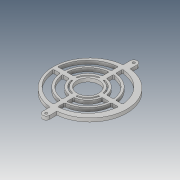
# Autodesk Inventor part: verticalThrusterCover2
Saved by Autodesk Inventor 2018 (Build 220112000, 112)
## iProperties
Created: 2020-02-09
Part Number: verticalThrusterCover2
Material: Generic
Document SubType Name: Modeling
Designer: anirudh
Density: 1 g/cm^3
Appearance: Default
Author: anirudh
Autodesk Inventor part; units mm, degrees
ref_plane "YZ Plane" through (0, 0, 0) normal (1, 0, 0) x (0, 1, 0)
ref_plane "XZ Plane" through (0, 0, 0) normal (0, 1, 0) x (-1, 0, 0)
ref_plane "XY Plane" through (0, 0, 0) normal (0, 0, 1) x (1, 0, 0)
sketch "Sketch1" plane through (0, 0, 0) normal (0, 1, 0) x (-1, 0, 0)
  circle A0 centre (0, -63.5) radius 1.75
  circle A1 centre (0, 63.5) radius 1.75
  circle A2 centre (0, -63.5) radius 1.75
  circle A3 centre (0, 63.5) radius 1.75
  arc A4 (5.08, 63.5) -> (-5.08, 63.5) centre (0, 63.5) ccw
  arc A5 (-5.08, -63.5) -> (5.08, -63.5) centre (0, -63.5) ccw
  line L0 (5.08, 63.5) -> (5.08, 53.0975)
  line L1 (5.08, -53.0975) -> (5.08, -63.5)
  line L2 (-5.08, -63.5) -> (-5.08, -53.0975)
  line L3 (-5.08, 53.0975) -> (-5.08, 63.5)
  arc A6 (-5.08, 53.0975) -> (-5.08, -53.0975) centre (0, 0) ccw
  arc A7 (5.08, -53.0975) -> (5.08, 53.0975) centre (0, 0) ccw
  arc A8 (-0.1848, -27.646) -> (6.1284, -27.646) centre (2.9718, -27.305) ccw
  line L4 (6.8199, -21.2443) -> (6.1284, -27.646)
  line L5 (-0.1848, -27.646) -> (-0.8763, -21.2443)
  line L6 (30.6178, -3.1566) -> (24.2161, -3.8481)
  line L7 (24.2161, 3.8481) -> (30.6178, 3.1566)
  arc A9 (30.6178, -3.1566) -> (30.6178, 3.1566) centre (30.2768, 0) ccw
  line L8 (6.1284, 27.646) -> (6.8199, 21.2443)
  line L9 (-0.8763, 21.2443) -> (-0.1848, 27.646)
  arc A10 (6.1284, 27.646) -> (-0.1848, 27.646) centre (2.9718, 27.305) ccw
  line L10 (-24.6742, 3.1566) -> (-18.2725, 3.8481)
  line L11 (-18.2725, -3.8481) -> (-24.6742, -3.1566)
  arc A11 (-24.6742, 3.1566) -> (-24.6742, -3.1566) centre (-24.3332, 0) ccw
  arc A12 (24.2161, 3.8481) -> (6.8199, 21.2443) centre (2.9718, 0) ccw
  arc A13 (-0.8763, 21.2443) -> (-18.2725, 3.8481) centre (2.9718, 0) ccw
  arc A14 (-18.2725, -3.8481) -> (-0.8763, -21.2443) centre (2.9718, 0) ccw
  arc A15 (6.8199, -21.2443) -> (24.2161, -3.8481) centre (2.9718, 0) ccw
  dimension "d34" = 360
  constraints: 24 end point, 24 point on circle, 16 centre point, 4 coincident, 4 vertical, 2 concentric, 33 other
extrude "Extrusion2" add sketch "Sketch1" along normal blind 5.08
sketch "Sketch3" plane through (0, 5.08, 0) normal (0, 1, 0) x (1, 0, 0)
  arc A0 (-6.8199, 21.2443) -> (-24.2161, 3.8481) centre (-2.9718, 0) ccw projected
  circle A1 centre (-2.9718, 0) radius 15.875
  circle A2 centre (-2.9718, 0) radius 38.7434
  point P0 (0, 0)
  dimension "d54" = 31.75
  constraints: 2 centre point, 2 coincident
  measures "d54" diameter of A1
extrude "Extrusion4" add sketch "Sketch3" against normal blind 5.08
sketch "Sketch4" plane through (0, 5.08, 0) normal (0, 1, 0) x (1, 0, 0)
  arc A0 (-50.0581, -3.175) -> (-6.1468, -47.0863) centre (-2.9718, 0) ccw
  arc A1 (0.2032, -47.0863) -> (44.1145, -3.175) centre (-2.9718, 0) ccw
  arc A2 (-40.0292, -3.175) -> (-6.1468, -37.0574) centre (-2.9718, 0) ccw
  arc A3 (0.2032, -37.0574) -> (34.0856, -3.175) centre (-2.9718, 0) ccw
  arc A4 (-36.8415, -3.175) -> (-6.1468, -33.8697) centre (-2.9718, 0) ccw
  arc A5 (0.2032, -33.8697) -> (30.8979, -3.175) centre (-2.9718, 0) ccw
  arc A6 (-26.7792, -3.175) -> (-6.1468, -23.8074) centre (-2.9718, 0) ccw
  arc A7 (0.2032, -23.8074) -> (20.8356, -3.175) centre (-2.9718, 0) ccw
  arc A8 (-23.5718, -3.175) -> (-6.1468, -20.6) centre (-2.9718, 0) ccw
  arc A9 (0.2032, -20.6) -> (17.6282, -3.175) centre (-2.9718, 0) ccw
  arc A10 (-21.7554, -3.175) -> (-6.1468, -18.7836) centre (-2.9718, 0) ccw
  arc A11 (0.2032, -18.7836) -> (15.8118, -3.175) centre (-2.9718, 0) ccw
  arc A12 (-21.7554, -3.175) -> (-6.1468, -18.7836) centre (-2.9718, 0) ccw
  arc A13 (0.2032, -18.7836) -> (15.8118, -3.175) centre (-2.9718, 0) ccw
  arc A14 (15.8118, 3.175) -> (0.2032, 18.7836) centre (-2.9718, 0) ccw
  arc A15 (-6.1468, 18.7836) -> (-21.7554, 3.175) centre (-2.9718, 0) ccw
  arc A16 (17.6282, 3.175) -> (0.2032, 20.6) centre (-2.9718, 0) ccw
  arc A17 (-6.1468, 20.6) -> (-23.5718, 3.175) centre (-2.9718, 0) ccw
  arc A18 (15.8118, 3.175) -> (0.2032, 18.7836) centre (-2.9718, 0) ccw
  arc A19 (-6.1468, 18.7836) -> (-21.7554, 3.175) centre (-2.9718, 0) ccw
  arc A20 (20.8356, 3.175) -> (0.2032, 23.8074) centre (-2.9718, 0) ccw
  arc A21 (-6.1468, 23.8074) -> (-26.7792, 3.175) centre (-2.9718, 0) ccw
  arc A22 (30.8979, 3.175) -> (0.2032, 33.8697) centre (-2.9718, 0) ccw
  arc A23 (-6.1468, 33.8697) -> (-36.8415, 3.175) centre (-2.9718, 0) ccw
  arc A24 (34.0856, 3.175) -> (0.2032, 37.0574) centre (-2.9718, 0) ccw
  arc A25 (-6.1468, 37.0574) -> (-40.0292, 3.175) centre (-2.9718, 0) ccw
  arc A26 (44.1145, 3.175) -> (0.2032, 47.0863) centre (-2.9718, 0) ccw
  arc A27 (-6.1468, 47.0863) -> (-50.0581, 3.175) centre (-2.9718, 0) ccw
  line L0 (-6.1468, -37.0574) -> (-6.1468, -47.0863)
  line L1 (0.2032, -37.0574) -> (0.2032, -47.0863)
  line L2 (-6.1468, -47.0863) -> (-6.1468, -37.0574)
  line L3 (-6.1468, -18.7836) -> (-6.1468, -20.6)
  line L4 (-6.1468, -23.8074) -> (-6.1468, -33.8697)
  line L5 (-6.1468, -33.8697) -> (-6.1468, -23.8074)
  line L6 (-6.1468, -20.6) -> (-6.1468, -18.7836)
  line L7 (0.2032, -18.7836) -> (0.2032, -20.6)
  line L8 (0.2032, -23.8074) -> (0.2032, -33.8697)
  line L9 (15.8118, -3.175) -> (17.6282, -3.175)
  line L10 (20.8356, -3.175) -> (30.8979, -3.175)
  line L11 (34.0856, -3.175) -> (44.1145, -3.175)
  line L12 (44.1145, 3.175) -> (34.0856, 3.175)
  line L13 (30.8979, 3.175) -> (20.8356, 3.175)
  line L14 (17.6282, 3.175) -> (15.8118, 3.175)
  line L15 (0.2032, 20.6) -> (0.2032, 18.7836)
  line L16 (0.2032, 47.0863) -> (0.2032, 37.0574)
  line L17 (0.2032, 33.8697) -> (0.2032, 23.8074)
  line L18 (-6.1468, 18.7836) -> (-6.1468, 20.6)
  line L19 (-6.1468, 23.8074) -> (-6.1468, 33.8697)
  line L20 (-6.1468, 37.0574) -> (-6.1468, 47.0863)
  line L21 (-21.7554, 3.175) -> (-23.5718, 3.175)
  line L22 (-26.7792, 3.175) -> (-36.8415, 3.175)
  line L23 (-40.0292, 3.175) -> (-50.0581, 3.175)
  line L24 (-40.0292, -3.175) -> (-50.0581, -3.175)
  line L25 (-21.7554, -3.175) -> (-23.5718, -3.175)
  line L26 (-26.7792, -3.175) -> (-36.8415, -3.175)
  constraints: 56 point on circle, 54 end point, 28 centre point, 7 coincident, 3 horizontal
extrude "Extrusion5" cut sketch "Sketch4" against normal blind 5.08
fillet "Fillet4" radius 1.27 32 edges at (-50.0581, 2.54, 3.175) (-40.0292, 2.54, 3.175) (-36.8415, 2.54, 3.175) (-26.7792, 2.54, 3.175) (-6.1468, 2.54, 47.0863) (-6.1468, 2.54, 37.0574) (-6.1468, 2.54, 33.8697) (-6.1468, 2.54, 23.8074) (0.2032, 2.54, 47.0863) (0.2032, 2.54, 37.0574) (0.2032, 2.54, 33.8697) (0.2032, 2.54, 23.8074) (20.8356, 2.54, 3.175) (30.8979, 2.54, 3.175) (34.0856, 2.54, 3.175) (44.1145, 2.54, 3.175) (44.1145, 2.54, -3.175) (34.0856, 2.54, -3.175) (30.8979, 2.54, -3.175) (20.8356, 2.54, -3.175) (0.2032, 2.54, -23.8074) (0.2032, 2.54, -33.8697) (0.2032, 2.54, -37.0574) (0.2032, 2.54, -47.0863) (-6.1468, 2.54, -23.8074) (-6.1468, 2.54, -33.8697) (-6.1468, 2.54, -37.0574) (-6.1468, 2.54, -47.0863) (-26.7792, 2.54, -3.175) (-50.0581, 2.54, -3.175) (-40.0292, 2.54, -3.175) (-36.8415, 2.54, -3.175)
fillet "Fillet5" radius 0.635 16 edges at (-23.5718, 2.54, 3.175) (-21.7554, 2.54, 3.175) (-6.1468, 2.54, 20.6) (-6.1468, 2.54, 18.7836) (0.2032, 2.54, 20.6) (0.2032, 2.54, 18.7836) (15.8118, 2.54, 3.175) (17.6282, 2.54, 3.175) (15.8118, 2.54, -3.175) (17.6282, 2.54, -3.175) (0.2032, 2.54, -18.7836) (0.2032, 2.54, -20.6) (-6.1468, 2.54, -18.7836) (-6.1468, 2.54, -20.6) (-23.5718, 2.54, -3.175) (-21.7554, 2.54, -3.175)
body "Solid2"
